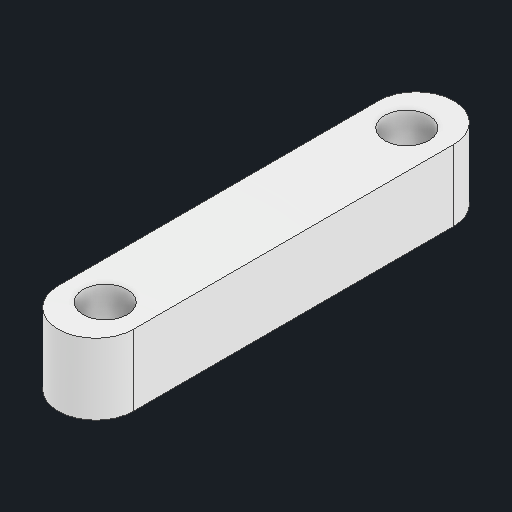
# Autodesk Inventor part: FourBarSection
Saved by Autodesk Inventor 2025 (Build 290162000, 162)
## iProperties
Created: 2024-05-20
Part Number: FourBarSection
Material: PC/ABS Plastic
Document SubType Name: Modeling
Designer: avsar
Density: 1.1 g/cm^3
Appearance: Smooth - White
Author: avsar
Autodesk Inventor part; units mm, degrees
ref_plane "YZ Plane" through (0, 0, 0) normal (1, 0, 0) x (0, 1, 0)
ref_plane "XZ Plane" through (0, 0, 0) normal (0, 1, 0) x (-1, 0, 0)
ref_plane "XY Plane" through (0, 0, 0) normal (0, 0, 1) x (1, 0, 0)
sketch "Sketch1" plane through (0, 0, 0) normal (0, 1, 0) x (-1, 0, 0)
  line L0 (6, 31.5) -> (-6, 31.5)
  line L1 (-6, 31.5) -> (-6, -31.5)
  line L2 (-6, -31.5) -> (6, -31.5)
  line L3 (6, -31.5) -> (6, 31.5)
  line L4 (6, 31.5) -> (-6, -31.5) construction
  line L5 (-6, 31.5) -> (6, -31.5) construction
  circle A0 centre (0, -24) radius 3.5
  line L6 (6, 0) -> (-6, 0) construction
  circle A1 centre (0, 24) radius 3.5
  point P0 (0, 0)
  dimension "d0" = 12
  dimension "d1" = 63
  dimension "d3" = 7
  dimension "d4" = 24
  constraints: 14 end point, 4 midpoint, 2 centre point, 2 parallel, 1 horizontal, 1 perpendicular, 1 symmetric about line, 1 vertical alignment, 1 other
  measures "d0" distance of L2.end L1.end
  measures "d1" distance of L0.end L1.end
  measures "d3" diameter of A0
  measures "d4" distance of A0.centre point (0, 0)
extrude "Extrusion1" add sketch "Sketch1" along normal blind 11.3
fillet "Fillet1" radius 6 4 edges at (-6, 5.65, 31.5) (6, 5.65, 31.5) (6, 5.65, -31.5) (-6, 5.65, -31.5)
body "Solid1"
